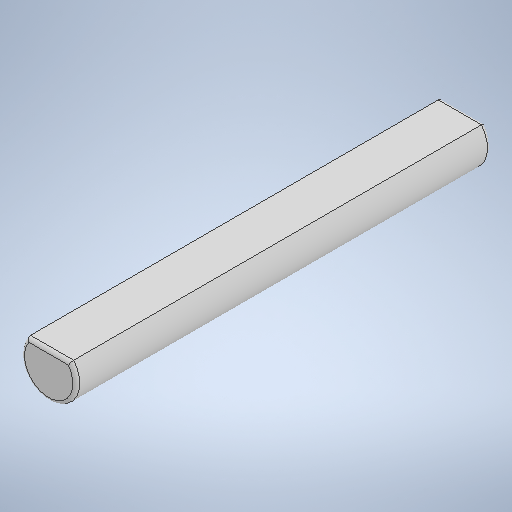
# Autodesk Inventor part: 8mm D-Shaft axle (3d print)
Saved by Autodesk Inventor 2025.3 (Build 293356030, 356C)
## iProperties
Created: 2025-10-10
Part Number: 8mm D-Shaft axle (3d print)
Material: Generic
Document SubType Name: Modeling
Designer: tvoko
Density: 1 g/cm^3
Appearance: Default
Author: tvoko
Autodesk Inventor part; units mm, degrees
ref_plane "YZ Plane" through (0, 0, 0) normal (1, 0, 0) x (0, 1, 0)
ref_plane "XZ Plane" through (0, 0, 0) normal (0, 1, 0) x (-1, 0, 0)
ref_plane "XY Plane" through (0, 0, 0) normal (0, 0, 1) x (1, 0, 0)
sketch "Sketch1" plane through (0, 0, 0) normal (0, 0, 1) x (1, 0, 0)
  circle A0 centre (0, 0) radius 4
  line L0 (-3.1225, 2.5) -> (3.1225, 2.5)
  dimension "d0" = 8
  dimension "d1" = 2.5
  constraints: 2 end point, 2 point on circle, 1 centre point, 1 coincident, 1 horizontal
  measures "d0" diameter of A0
  measures "d1" distance from line of L0 point (0, 0)
extrude "Extrusion1" add sketch "Sketch1" along normal blind 60 contours A0 L0 picked at (-0.7341, 0.0257)
fillet "Fillet1" radius 0.5 4 edges at (0, -4, 60) (0, 2.5, 60) (0, -4, 0) (0, 2.5, 0)
body "Solid1"
